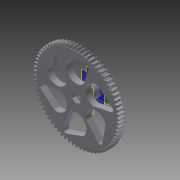
# Autodesk Inventor part: quarterinch-gear2
Saved by Autodesk Inventor 2014 (Build 180170000, 170)
## iProperties
Created: 2013-11-06
Part Number: quarterinch-gear2
Material: Generic
Document SubType Name: Modeling
Designer: stephen
Density: 1 g/cm^3
Appearance: Default
Author: stephen
Autodesk Inventor part; units mm, degrees
ref_plane "YZ Plane" through (0, 0, 0) normal (1, 0, 0) x (0, 1, 0)
ref_plane "XZ Plane" through (0, 0, 0) normal (0, 1, 0) x (-1, 0, 0)
ref_plane "XY Plane" through (0, 0, 0) normal (0, 0, 1) x (1, 0, 0)
ref_plane "Work Plane10" through (2.7665, 46.0619, 25.38) normal (0, 0, 1) x (1, 0, 0)
sketch "Sketch15" plane through (2.7665, 46.0619, 25.38) normal (0, 0, 1) x (1, 0, 0)
  line L0 (-0.1767, 42.3028) -> (0.1689, 42.3028)
  arc A0 (0.9579, 39.3583) -> (0.1689, 42.3028) centre (-2.8295, 39.9215) ccw
  line L1 (0.1689, 42.3028) -> (0.9579, 39.3583) construction
  arc A1 (-0.1767, 42.3028) -> (-0.9656, 39.3582) centre (2.8217, 39.9215) ccw
  line L2 (-3.968, 42.1167) -> (-3.6238, 42.1476)
  arc A2 (-2.5741, 39.2858) -> (-3.6238, 42.1476) centre (-6.3966, 39.5071) ccw
  line L3 (-3.6238, 42.1476) -> (-2.5741, 39.2858) construction
  arc A3 (-3.968, 42.1167) -> (-4.4898, 39.1132) centre (-0.7682, 40.0137) ccw
  line L4 (-7.7273, 41.5914) -> (-7.3873, 41.6531)
  arc A4 (-6.0852, 38.8969) -> (-7.3873, 41.6531) centre (-9.9122, 38.7747) ccw
  line L5 (-7.3873, 41.6531) -> (-6.0852, 38.8969) construction
  arc A5 (-7.7273, 41.5914) -> (-7.9778, 38.5532) centre (-4.3519, 39.7837) ccw
  line L6 (-11.4244, 40.7313) -> (-11.0913, 40.8233)
  arc A6 (-9.5474, 38.1948) -> (-11.0913, 40.8233) centre (-13.3481, 37.7301) ccw
  line L7 (-11.0913, 40.8233) -> (-9.5474, 38.1948) construction
  arc A7 (-11.4244, 40.7313) -> (-11.4015, 37.6829) centre (-7.9006, 39.2335) ccw
  line L8 (-15.0295, 39.5433) -> (-14.706, 39.6647)
  arc A8 (-12.9328, 37.1852) -> (-14.706, 39.6647) centre (-16.6764, 36.3817) ccw
  line L9 (-14.706, 39.6647) -> (-12.9328, 37.1852) construction
  arc A9 (-15.0295, 39.5433) -> (-14.7335, 36.5092) centre (-11.3856, 38.3673) ccw
  line L10 (-18.5137, 38.0368) -> (-18.2023, 38.1868)
  arc A10 (-16.2139, 35.8762) -> (-18.2023, 38.1868) centre (-19.8705, 34.7403) ccw
  line L11 (-18.2023, 38.1868) -> (-16.2139, 35.8762) construction
  arc A11 (-18.5137, 38.0368) -> (-17.9468, 35.0415) centre (-14.779, 37.1923) ccw
  line L12 (-21.8487, 36.2242) -> (-21.5521, 36.4014)
  arc A12 (-19.3646, 34.2784) -> (-21.5521, 36.4014) centre (-22.9046, 32.8193) ccw
  line L13 (-21.5521, 36.4014) -> (-19.3646, 34.2784) construction
  arc A13 (-21.8487, 36.2242) -> (-21.0157, 33.2917) centre (-18.0534, 35.7178) ccw
  line L14 (-25.0079, 34.1198) -> (-24.7283, 34.323)
  arc A14 (-22.3593, 32.4046) -> (-24.7283, 34.323) centre (-25.7543, 30.634) ccw
  line L15 (-24.7283, 34.323) -> (-22.3593, 32.4046) construction
  arc A15 (-25.0079, 34.1198) -> (-23.9153, 31.2738) centre (-21.1825, 33.9557) ccw
  line L16 (-27.9657, 31.7408) -> (-27.7055, 31.9681)
  arc A16 (-25.174, 30.2699) -> (-27.7055, 31.9681) centre (-28.3967, 28.2021) ccw
  line L17 (-27.7055, 31.9681) -> (-25.174, 30.2699) construction
  arc A17 (-27.9657, 31.7408) -> (-26.6224, 29.0042) centre (-24.1409, 31.9202) ccw
  line L18 (-30.6983, 29.1062) -> (-30.4595, 29.356)
  arc A18 (-27.7861, 27.8914) -> (-30.4595, 29.356) centre (-30.8104, 25.5431) ccw
  line L19 (-30.4595, 29.356) -> (-27.7861, 27.8914) construction
  arc A19 (-30.6983, 29.1062) -> (-29.1152, 26.501) centre (-26.9051, 29.6277) ccw
  line L20 (-33.1838, 26.2372) -> (-32.9683, 26.5074)
  arc A20 (-30.1744, 25.2884) -> (-32.9683, 26.5074) centre (-32.976, 22.6785) ccw
  line L21 (-32.9683, 26.5074) -> (-30.1744, 25.2884) construction
  arc A21 (-33.1838, 26.2372) -> (-31.3735, 23.7845) centre (-29.4526, 27.0967) ccw
  line L22 (-35.4021, 23.157) -> (-35.2117, 23.4454)
  arc A22 (-32.3197, 22.4818) -> (-35.2117, 23.4454) centre (-34.8761, 19.6312) ccw
  line L23 (-35.2117, 23.4454) -> (-32.3197, 22.4818) construction
  arc A23 (-35.4021, 23.157) -> (-33.3792, 20.8764) centre (-31.7629, 24.3475) ccw
  line L24 (-37.3354, 19.8904) -> (-37.1716, 20.1947)
  arc A24 (-34.2049, 19.4942) -> (-37.1716, 20.1947) centre (-36.4955, 16.4259) ccw
  line L25 (-37.1716, 20.1947) -> (-34.2049, 19.4942) construction
  arc A25 (-37.3354, 19.8904) -> (-35.1162, 17.8003) centre (-33.8176, 21.4023) ccw
  line L26 (-38.968, 16.4636) -> (-38.8322, 16.7814)
  arc A26 (-35.8146, 16.3496) -> (-38.8322, 16.7814) centre (-37.8209, 13.0884) ccw
  line L27 (-38.8322, 16.7814) -> (-35.8146, 16.3496) construction
  arc A27 (-38.968, 16.4636) -> (-36.5704, 14.5808) centre (-35.5999, 18.2847) ccw
  line L28 (-40.2869, 12.9043) -> (-40.1802, 13.2329)
  arc A28 (-37.136, 13.0734) -> (-40.1802, 13.2329) centre (-38.8419, 9.6454) ccw
  line L29 (-40.1802, 13.2329) -> (-37.136, 13.0734) construction
  arc A29 (-40.2869, 12.9043) -> (-37.7302, 11.244) centre (-37.0956, 15.02) ccw
  line L30 (-41.2815, 9.241) -> (-41.2046, 9.5779)
  arc A30 (-38.1584, 9.6919) -> (-41.2046, 9.5779) centre (-39.5502, 6.1248) ccw
  line L31 (-41.2046, 9.5779) -> (-38.1584, 9.6919) construction
  arc A31 (-41.2815, 9.241) -> (-38.5862, 7.8166) centre (-38.2927, 11.6343) ccw
  line L32 (-41.9437, 5.5034) -> (-41.8973, 5.8458)
  arc A32 (-38.8736, 6.2324) -> (-41.8973, 5.8458) centre (-39.94, 2.5549) ccw
  line L33 (-41.8973, 5.8458) -> (-38.8736, 6.2324) construction
  arc A33 (-41.9437, 5.5034) -> (-39.1316, 4.3263) centre (-39.1814, 8.1549) ccw
  line L34 (-42.2681, 1.7214) -> (-42.2526, 2.0666)
  arc A34 (-39.2757, 2.7227) -> (-42.2526, 2.0666) centre (-40.0082, -1.0355) ccw
  line L35 (-42.2526, 2.0666) -> (-39.2757, 2.7227) construction
  arc A35 (-42.2681, 1.7214) -> (-39.3618, 0.8012) centre (-39.7547, 4.6099) ccw
  line L36 (-42.2523, -2.0744) -> (-42.2678, -1.7292)
  arc A36 (-39.3617, -0.8089) -> (-42.2678, -1.7292) centre (-39.7543, -4.6177) ccw
  line L37 (-42.2678, -1.7292) -> (-39.3617, -0.8089) construction
  arc A37 (-42.2523, -2.0744) -> (-39.2752, -2.7304) centre (-40.0079, 1.0278) ccw
  line L38 (-41.8962, -5.8535) -> (-41.9426, -5.5111)
  arc A38 (-39.1307, -4.334) -> (-41.9426, -5.5111) centre (-39.1804, -8.1626) ccw
  line L39 (-41.9426, -5.5111) -> (-39.1307, -4.334) construction
  arc A39 (-41.8962, -5.8535) -> (-38.8723, -6.24) centre (-39.9389, -2.5626) ccw
  line L40 (-41.2029, -9.5855) -> (-41.2798, -9.2486)
  arc A40 (-38.5847, -7.8242) -> (-41.2798, -9.2486) centre (-38.2909, -11.6419) ccw
  line L41 (-41.2798, -9.2486) -> (-38.5847, -7.8242) construction
  arc A41 (-41.2029, -9.5855) -> (-38.1565, -9.6994) centre (-39.5484, -6.1324) ccw
  line L42 (-40.1777, -13.2403) -> (-40.2845, -12.9117)
  arc A42 (-37.728, -11.2514) -> (-40.2845, -12.9117) centre (-37.0932, -15.0274) ccw
  line L43 (-40.2845, -12.9117) -> (-37.728, -11.2514) construction
  arc A43 (-40.1777, -13.2403) -> (-37.1334, -13.0807) centre (-38.8395, -9.6528) ccw
  line L44 (-38.8292, -16.7885) -> (-38.965, -16.4708)
  arc A44 (-36.5676, -14.588) -> (-38.965, -16.4708) centre (-35.5968, -18.2919) ccw
  line L45 (-38.965, -16.4708) -> (-36.5676, -14.588) construction
  arc A45 (-38.8292, -16.7885) -> (-35.8114, -16.3566) centre (-37.8179, -13.0955) ccw
  line L46 (-37.1679, -20.2015) -> (-37.3317, -19.8972)
  arc A46 (-35.1127, -17.8072) -> (-37.3317, -19.8972) centre (-33.8139, -21.4091) ccw
  line L47 (-37.3317, -19.8972) -> (-35.1127, -17.8072) construction
  arc A47 (-37.1679, -20.2015) -> (-34.201, -19.5009) centre (-36.4918, -16.4328) ccw
  line L48 (-35.2074, -23.4519) -> (-35.3978, -23.1635)
  arc A48 (-33.3751, -20.883) -> (-35.3978, -23.1635) centre (-31.7586, -24.354) ccw
  line L49 (-35.3978, -23.1635) -> (-33.3751, -20.883) construction
  arc A49 (-35.2074, -23.4519) -> (-32.3153, -22.4882) centre (-34.8718, -19.6377) ccw
  line L50 (-32.9635, -26.5135) -> (-33.179, -26.2433)
  arc A50 (-31.3688, -23.7906) -> (-33.179, -26.2433) centre (-29.4477, -27.1028) ccw
  line L51 (-33.179, -26.2433) -> (-31.3688, -23.7906) construction
  arc A51 (-32.9635, -26.5135) -> (-30.1694, -25.2944) centre (-32.9711, -22.6845) ccw
  line L52 (-30.4541, -29.3616) -> (-30.693, -29.1118)
  arc A52 (-29.1099, -26.5067) -> (-30.693, -29.1118) centre (-26.8997, -29.6333) ccw
  line L53 (-30.693, -29.1118) -> (-29.1099, -26.5067) construction
  arc A53 (-30.4541, -29.3616) -> (-27.7806, -27.8969) centre (-30.805, -25.5487) ccw
  line L54 (-27.6996, -31.9733) -> (-27.9598, -31.7459)
  arc A54 (-26.6167, -29.0094) -> (-27.9598, -31.7459) centre (-24.1351, -31.9253) ccw
  line L55 (-27.9598, -31.7459) -> (-26.6167, -29.0094) construction
  arc A55 (-27.6996, -31.9733) -> (-25.1681, -30.2748) centre (-28.3908, -28.2072) ccw
  line L56 (-24.722, -34.3275) -> (-25.0016, -34.1244)
  arc A56 (-23.9092, -31.2786) -> (-25.0016, -34.1244) centre (-21.1762, -33.9603) ccw
  line L57 (-25.0016, -34.1244) -> (-23.9092, -31.2786) construction
  arc A57 (-24.722, -34.3275) -> (-22.3529, -32.409) centre (-25.748, -30.6386) ccw
  line L58 (-21.5454, -36.4054) -> (-21.8421, -36.2282)
  arc A58 (-21.0091, -33.2958) -> (-21.8421, -36.2282) centre (-18.0467, -35.7218) ccw
  line L59 (-21.8421, -36.2282) -> (-21.0091, -33.2958) construction
  arc A59 (-21.5454, -36.4054) -> (-19.3578, -34.2822) centre (-22.898, -32.8233) ccw
  line L60 (-18.1953, -38.1902) -> (-18.5067, -38.0402)
  arc A60 (-17.9399, -35.045) -> (-18.5067, -38.0402) centre (-14.772, -37.1956) ccw
  line L61 (-18.5067, -38.0402) -> (-17.9399, -35.045) construction
  arc A61 (-18.1953, -38.1902) -> (-16.2069, -35.8794) centre (-19.8635, -34.7437) ccw
  line L62 (-14.6987, -39.6674) -> (-15.0223, -39.546)
  arc A62 (-14.7263, -36.5121) -> (-15.0223, -39.546) centre (-11.3784, -38.3701) ccw
  line L63 (-15.0223, -39.546) -> (-14.7263, -36.5121) construction
  arc A63 (-14.6987, -39.6674) -> (-12.9254, -37.1878) centre (-16.6692, -36.3844) ccw
  line L64 (-11.0838, -40.8253) -> (-11.4169, -40.7334)
  arc A64 (-11.3941, -37.6852) -> (-11.4169, -40.7334) centre (-7.8931, -39.2355) ccw
  line L65 (-11.4169, -40.7334) -> (-11.3941, -37.6852) construction
  arc A65 (-11.0838, -40.8253) -> (-9.5399, -38.1967) centre (-13.3406, -37.7321) ccw
  line L66 (-7.3796, -41.6545) -> (-7.7196, -41.5928)
  arc A66 (-7.9702, -38.5548) -> (-7.7196, -41.5928) centre (-4.3443, -39.7851) ccw
  line L67 (-7.7196, -41.5928) -> (-7.9702, -38.5548) construction
  arc A67 (-7.3796, -41.6545) -> (-6.0776, -38.8981) centre (-9.9046, -38.7761) ccw
  line L68 (-3.616, -42.1483) -> (-3.9602, -42.1174)
  arc A68 (-4.4821, -39.114) -> (-3.9602, -42.1174) centre (-0.7605, -40.0144) ccw
  line L69 (-3.9602, -42.1174) -> (-4.4821, -39.114) construction
  arc A69 (-3.616, -42.1483) -> (-2.5663, -39.2863) centre (-6.3889, -39.5078) ccw
  line L70 (0.1767, -42.3028) -> (-0.1689, -42.3028)
  arc A70 (-0.9579, -39.3583) -> (-0.1689, -42.3028) centre (2.8295, -39.9215) ccw
  line L71 (-0.1689, -42.3028) -> (-0.9579, -39.3583) construction
  arc A71 (0.1767, -42.3028) -> (0.9656, -39.3582) centre (-2.8217, -39.9215) ccw
  line L72 (3.968, -42.1167) -> (3.6238, -42.1476)
  arc A72 (2.5741, -39.2858) -> (3.6238, -42.1476) centre (6.3966, -39.5071) ccw
  line L73 (3.6238, -42.1476) -> (2.5741, -39.2858) construction
  arc A73 (3.968, -42.1167) -> (4.4898, -39.1132) centre (0.7682, -40.0137) ccw
  line L74 (7.7273, -41.5914) -> (7.3873, -41.6531)
  arc A74 (6.0852, -38.8969) -> (7.3873, -41.6531) centre (9.9122, -38.7747) ccw
  line L75 (7.3873, -41.6531) -> (6.0852, -38.8969) construction
  arc A75 (7.7273, -41.5914) -> (7.9778, -38.5532) centre (4.3519, -39.7837) ccw
  line L76 (11.4244, -40.7313) -> (11.0913, -40.8233)
  arc A76 (9.5474, -38.1948) -> (11.0913, -40.8233) centre (13.3481, -37.7301) ccw
  line L77 (11.0913, -40.8233) -> (9.5474, -38.1948) construction
  arc A77 (11.4244, -40.7313) -> (11.4015, -37.6829) centre (7.9006, -39.2335) ccw
  line L78 (15.0295, -39.5433) -> (14.706, -39.6647)
  arc A78 (12.9328, -37.1852) -> (14.706, -39.6647) centre (16.6764, -36.3817) ccw
  line L79 (14.706, -39.6647) -> (12.9328, -37.1852) construction
  arc A79 (15.0295, -39.5433) -> (14.7335, -36.5092) centre (11.3856, -38.3673) ccw
  line L80 (18.5137, -38.0368) -> (18.2023, -38.1868)
  arc A80 (16.2139, -35.8762) -> (18.2023, -38.1868) centre (19.8705, -34.7403) ccw
  line L81 (18.2023, -38.1868) -> (16.2139, -35.8762) construction
  arc A81 (18.5137, -38.0368) -> (17.9468, -35.0415) centre (14.779, -37.1923) ccw
  line L82 (21.8487, -36.2242) -> (21.5521, -36.4014)
  arc A82 (19.3646, -34.2784) -> (21.5521, -36.4014) centre (22.9046, -32.8193) ccw
  line L83 (21.5521, -36.4014) -> (19.3646, -34.2784) construction
  arc A83 (21.8487, -36.2242) -> (21.0157, -33.2917) centre (18.0534, -35.7178) ccw
  line L84 (25.0079, -34.1198) -> (24.7283, -34.323)
  arc A84 (22.3593, -32.4046) -> (24.7283, -34.323) centre (25.7543, -30.634) ccw
  line L85 (24.7283, -34.323) -> (22.3593, -32.4046) construction
  arc A85 (25.0079, -34.1198) -> (23.9153, -31.2738) centre (21.1825, -33.9557) ccw
  line L86 (27.9657, -31.7408) -> (27.7055, -31.9681)
  arc A86 (25.174, -30.2699) -> (27.7055, -31.9681) centre (28.3967, -28.2021) ccw
  line L87 (27.7055, -31.9681) -> (25.174, -30.2699) construction
  arc A87 (27.9657, -31.7408) -> (26.6224, -29.0042) centre (24.1409, -31.9202) ccw
  line L88 (30.6983, -29.1062) -> (30.4595, -29.356)
  arc A88 (27.7861, -27.8914) -> (30.4595, -29.356) centre (30.8104, -25.5431) ccw
  line L89 (30.4595, -29.356) -> (27.7861, -27.8914) construction
  arc A89 (30.6983, -29.1062) -> (29.1152, -26.501) centre (26.9051, -29.6277) ccw
  line L90 (33.1838, -26.2372) -> (32.9683, -26.5074)
  arc A90 (30.1744, -25.2884) -> (32.9683, -26.5074) centre (32.976, -22.6785) ccw
  line L91 (32.9683, -26.5074) -> (30.1744, -25.2884) construction
  arc A91 (33.1838, -26.2372) -> (31.3735, -23.7845) centre (29.4526, -27.0967) ccw
  line L92 (35.4021, -23.157) -> (35.2117, -23.4454)
  arc A92 (32.3197, -22.4818) -> (35.2117, -23.4454) centre (34.8761, -19.6312) ccw
  line L93 (35.2117, -23.4454) -> (32.3197, -22.4818) construction
  arc A93 (35.4021, -23.157) -> (33.3792, -20.8764) centre (31.7629, -24.3475) ccw
  line L94 (37.3354, -19.8904) -> (37.1716, -20.1947)
  arc A94 (34.2049, -19.4942) -> (37.1716, -20.1947) centre (36.4955, -16.4259) ccw
  line L95 (37.1716, -20.1947) -> (34.2049, -19.4942) construction
  arc A95 (37.3354, -19.8904) -> (35.1162, -17.8003) centre (33.8176, -21.4023) ccw
  line L96 (38.968, -16.4636) -> (38.8322, -16.7814)
  arc A96 (35.8146, -16.3496) -> (38.8322, -16.7814) centre (37.8209, -13.0884) ccw
  line L97 (38.8322, -16.7814) -> (35.8146, -16.3496) construction
  arc A97 (38.968, -16.4636) -> (36.5704, -14.5808) centre (35.5999, -18.2847) ccw
  line L98 (40.2869, -12.9043) -> (40.1802, -13.2329)
  arc A98 (37.136, -13.0734) -> (40.1802, -13.2329) centre (38.8419, -9.6454) ccw
  line L99 (40.1802, -13.2329) -> (37.136, -13.0734) construction
  arc A99 (40.2869, -12.9043) -> (37.7302, -11.244) centre (37.0956, -15.02) ccw
  line L100 (41.2815, -9.241) -> (41.2046, -9.5779)
  arc A100 (38.1584, -9.6919) -> (41.2046, -9.5779) centre (39.5502, -6.1248) ccw
  line L101 (41.2046, -9.5779) -> (38.1584, -9.6919) construction
  arc A101 (41.2815, -9.241) -> (38.5862, -7.8166) centre (38.2927, -11.6343) ccw
  line L102 (41.9437, -5.5034) -> (41.8973, -5.8458)
  arc A102 (38.8736, -6.2324) -> (41.8973, -5.8458) centre (39.94, -2.5549) ccw
  line L103 (41.8973, -5.8458) -> (38.8736, -6.2324) construction
  arc A103 (41.9437, -5.5034) -> (39.1316, -4.3263) centre (39.1814, -8.1549) ccw
  line L104 (42.2681, -1.7214) -> (42.2526, -2.0666)
  arc A104 (39.2757, -2.7227) -> (42.2526, -2.0666) centre (40.0082, 1.0355) ccw
  line L105 (42.2526, -2.0666) -> (39.2757, -2.7227) construction
  arc A105 (42.2681, -1.7214) -> (39.3618, -0.8012) centre (39.7547, -4.6099) ccw
  line L106 (42.2523, 2.0744) -> (42.2678, 1.7292)
  arc A106 (39.3617, 0.8089) -> (42.2678, 1.7292) centre (39.7543, 4.6177) ccw
  line L107 (42.2678, 1.7292) -> (39.3617, 0.8089) construction
  arc A107 (42.2523, 2.0744) -> (39.2752, 2.7304) centre (40.0079, -1.0278) ccw
  line L108 (41.8962, 5.8535) -> (41.9426, 5.5111)
  arc A108 (39.1307, 4.334) -> (41.9426, 5.5111) centre (39.1804, 8.1626) ccw
  line L109 (41.9426, 5.5111) -> (39.1307, 4.334) construction
  arc A109 (41.8962, 5.8535) -> (38.8723, 6.24) centre (39.9389, 2.5626) ccw
  line L110 (41.2029, 9.5855) -> (41.2798, 9.2486)
  arc A110 (38.5847, 7.8242) -> (41.2798, 9.2486) centre (38.2909, 11.6419) ccw
  line L111 (41.2798, 9.2486) -> (38.5847, 7.8242) construction
  arc A111 (41.2029, 9.5855) -> (38.1565, 9.6994) centre (39.5484, 6.1324) ccw
  line L112 (40.1777, 13.2403) -> (40.2845, 12.9117)
  arc A112 (37.728, 11.2514) -> (40.2845, 12.9117) centre (37.0932, 15.0274) ccw
  line L113 (40.2845, 12.9117) -> (37.728, 11.2514) construction
  arc A113 (40.1777, 13.2403) -> (37.1334, 13.0807) centre (38.8395, 9.6528) ccw
  line L114 (38.8292, 16.7885) -> (38.965, 16.4708)
  arc A114 (36.5676, 14.588) -> (38.965, 16.4708) centre (35.5968, 18.2919) ccw
  line L115 (38.965, 16.4708) -> (36.5676, 14.588) construction
  arc A115 (38.8292, 16.7885) -> (35.8114, 16.3566) centre (37.8179, 13.0955) ccw
  line L116 (37.1679, 20.2015) -> (37.3317, 19.8972)
  arc A116 (35.1127, 17.8072) -> (37.3317, 19.8972) centre (33.8139, 21.4091) ccw
  line L117 (37.3317, 19.8972) -> (35.1127, 17.8072) construction
  arc A117 (37.1679, 20.2015) -> (34.201, 19.5009) centre (36.4918, 16.4328) ccw
  line L118 (35.2074, 23.4519) -> (35.3978, 23.1635)
  arc A118 (33.3751, 20.883) -> (35.3978, 23.1635) centre (31.7586, 24.354) ccw
  line L119 (35.3978, 23.1635) -> (33.3751, 20.883) construction
  arc A119 (35.2074, 23.4519) -> (32.3153, 22.4882) centre (34.8718, 19.6377) ccw
  line L120 (32.9635, 26.5135) -> (33.179, 26.2433)
  arc A120 (31.3688, 23.7906) -> (33.179, 26.2433) centre (29.4477, 27.1028) ccw
  line L121 (33.179, 26.2433) -> (31.3688, 23.7906) construction
  arc A121 (32.9635, 26.5135) -> (30.1694, 25.2944) centre (32.9711, 22.6845) ccw
  line L122 (30.4541, 29.3616) -> (30.693, 29.1118)
  arc A122 (29.1099, 26.5067) -> (30.693, 29.1118) centre (26.8997, 29.6333) ccw
  line L123 (30.693, 29.1118) -> (29.1099, 26.5067) construction
  arc A123 (30.4541, 29.3616) -> (27.7806, 27.8969) centre (30.805, 25.5487) ccw
  line L124 (27.6996, 31.9733) -> (27.9598, 31.7459)
  arc A124 (26.6167, 29.0094) -> (27.9598, 31.7459) centre (24.1351, 31.9253) ccw
  line L125 (27.9598, 31.7459) -> (26.6167, 29.0094) construction
  arc A125 (27.6996, 31.9733) -> (25.1681, 30.2748) centre (28.3908, 28.2072) ccw
  line L126 (24.722, 34.3275) -> (25.0016, 34.1244)
  arc A126 (23.9092, 31.2786) -> (25.0016, 34.1244) centre (21.1762, 33.9603) ccw
  line L127 (25.0016, 34.1244) -> (23.9092, 31.2786) construction
  arc A127 (24.722, 34.3275) -> (22.3529, 32.409) centre (25.748, 30.6386) ccw
  line L128 (21.5454, 36.4054) -> (21.8421, 36.2282)
  arc A128 (21.0091, 33.2958) -> (21.8421, 36.2282) centre (18.0467, 35.7218) ccw
  line L129 (21.8421, 36.2282) -> (21.0091, 33.2958) construction
  arc A129 (21.5454, 36.4054) -> (19.3578, 34.2822) centre (22.898, 32.8233) ccw
  line L130 (18.1953, 38.1902) -> (18.5067, 38.0402)
  arc A130 (17.9399, 35.045) -> (18.5067, 38.0402) centre (14.772, 37.1956) ccw
  line L131 (18.5067, 38.0402) -> (17.9399, 35.045) construction
  arc A131 (18.1953, 38.1902) -> (16.2069, 35.8794) centre (19.8635, 34.7437) ccw
  line L132 (14.6987, 39.6674) -> (15.0223, 39.546)
  arc A132 (14.7263, 36.5121) -> (15.0223, 39.546) centre (11.3784, 38.3701) ccw
  line L133 (15.0223, 39.546) -> (14.7263, 36.5121) construction
  arc A133 (14.6987, 39.6674) -> (12.9254, 37.1878) centre (16.6692, 36.3844) ccw
  line L134 (11.0838, 40.8253) -> (11.4169, 40.7334)
  arc A134 (11.3941, 37.6852) -> (11.4169, 40.7334) centre (7.8931, 39.2355) ccw
  line L135 (11.4169, 40.7334) -> (11.3941, 37.6852) construction
  arc A135 (11.0838, 40.8253) -> (9.5399, 38.1967) centre (13.3406, 37.7321) ccw
  line L136 (7.3796, 41.6545) -> (7.7196, 41.5928)
  arc A136 (7.9702, 38.5548) -> (7.7196, 41.5928) centre (4.3443, 39.7851) ccw
  line L137 (7.7196, 41.5928) -> (7.9702, 38.5548) construction
  arc A137 (7.3796, 41.6545) -> (6.0776, 38.8981) centre (9.9046, 38.7761) ccw
  line L138 (3.616, 42.1483) -> (3.9602, 42.1174)
  arc A138 (4.4821, 39.114) -> (3.9602, 42.1174) centre (0.7605, 40.0144) ccw
  line L139 (3.9602, 42.1174) -> (4.4821, 39.114) construction
  arc A139 (3.616, 42.1483) -> (2.5663, 39.2863) centre (6.3889, 39.5078) ccw
  line L140 (73.0043, -23.5061) -> (73.0043, 76.8994)
  line L141 (73.0043, -23.5061) -> (-27.4013, -23.5061) construction
  line L142 (12.7685, 31.9695) -> (7.0232, 15.0428)
  line L143 (-7.0232, 29.0892) -> (9.6761, 35.0189)
  arc A140 (-7.0232, 29.0892) -> (7.0232, 15.0428) centre (0, 22.066) ccw
  arc A141 (12.7685, 31.9695) -> (9.6761, 35.0189) centre (10.4835, 32.745) ccw
  line L144 (34.1169, 4.9001) -> (16.5854, 1.4124)
  arc A142 (21.7267, 20.6) -> (16.5854, 1.4124) centre (19.1561, 11.0062) ccw
  line L145 (21.7267, 20.6) -> (35.2117, 9.103)
  arc A143 (34.1169, 4.9001) -> (35.2117, 9.103) centre (33.6461, 7.2667) ccw
  line L146 (21.3176, -27.0693) -> (9.5313, -13.6305)
  arc A144 (28.719, -8.4891) -> (9.5313, -13.6305) centre (19.1252, -11.0598) ccw
  line L147 (28.719, -8.4891) -> (25.5047, -25.916)
  arc A145 (21.3176, -27.0693) -> (25.5047, -25.916) centre (23.1317, -25.4783) ccw
  line L148 (-12.7685, -31.9695) -> (-7.0232, -15.0428)
  arc A146 (7.0232, -29.0892) -> (-7.0232, -15.0428) centre (0, -22.066) ccw
  line L149 (7.0232, -29.0892) -> (-9.6761, -35.0189)
  arc A147 (-12.7685, -31.9695) -> (-9.6761, -35.0189) centre (-10.4835, -32.745) ccw
  line L150 (-34.0551, -4.9002) -> (-16.5236, -1.4124)
  arc A148 (-21.6649, -20.6001) -> (-16.5236, -1.4124) centre (-19.0942, -11.0062) ccw
  line L151 (-21.6649, -20.6001) -> (-35.1498, -9.103)
  arc A149 (-34.0551, -4.9002) -> (-35.1498, -9.103) centre (-33.5843, -7.2668) ccw
  line L152 (-21.2557, 27.0693) -> (-9.4695, 13.6304)
  arc A150 (-28.6572, 8.489) -> (-9.4695, 13.6304) centre (-19.0633, 11.0597) ccw
  line L153 (-28.6572, 8.489) -> (-25.4429, 25.9159)
  arc A151 (-21.2557, 27.0693) -> (-25.4429, 25.9159) centre (-23.0699, 25.4782) ccw
  line L154 (11.0838, 0) -> (38.8367, 0) construction
  line L155 (0, 0) -> (0, -16.4636)
  line L156 (0, 0) -> (9.5313, 0)
  line L157 (11.0838, 0) -> (9.4861, 0)
  line L158 (2.4848, 0) -> (0, 0)
  line L159 (0, 0) -> (0, -5.6488)
  line L160 (0, -11.1197) -> (0, -12.1337)
  arc A152 (-32.3153, -22.4882) -> (-31.3688, -23.7906) centre (0, 0) ccw
  arc A153 (-34.201, -19.5009) -> (-33.3751, -20.883) centre (0, 0) ccw
  arc A154 (-35.8114, -16.3566) -> (-35.1127, -17.8072) centre (0, 0) ccw
  arc A155 (-37.1334, -13.0807) -> (-36.5676, -14.588) centre (0, 0) ccw
  arc A156 (-38.8723, -6.24) -> (-38.5847, -7.8242) centre (0, 0) ccw
  arc A157 (-38.1565, -9.6994) -> (-37.728, -11.2514) centre (0, 0) ccw
  arc A158 (-39.2752, -2.7304) -> (-39.1307, -4.334) centre (0, 0) ccw
  arc A159 (-39.3618, 0.8012) -> (-39.3617, -0.8089) centre (0, 0) ccw
  arc A160 (-39.1316, 4.3263) -> (-39.2757, 2.7227) centre (0, 0) ccw
  arc A161 (-38.5862, 7.8166) -> (-38.8736, 6.2324) centre (0, 0) ccw
  arc A162 (-37.7302, 11.244) -> (-38.1584, 9.6919) centre (0, 0) ccw
  arc A163 (-36.5704, 14.5808) -> (-37.136, 13.0734) centre (0, 0) ccw
  arc A164 (-35.1162, 17.8003) -> (-35.8146, 16.3496) centre (0, 0) ccw
  arc A165 (-30.1694, -25.2944) -> (-29.1099, -26.5067) centre (0, 0) ccw
  arc A166 (-27.7806, -27.8969) -> (-26.6167, -29.0094) centre (0, 0) ccw
  arc A167 (-25.1681, -30.2748) -> (-23.9092, -31.2786) centre (0, 0) ccw
  arc A168 (-22.3529, -32.409) -> (-21.0091, -33.2958) centre (0, 0) ccw
  arc A169 (-19.3578, -34.2822) -> (-17.9399, -35.045) centre (0, 0) ccw
  arc A170 (-16.2069, -35.8794) -> (-14.7263, -36.5121) centre (0, 0) ccw
  arc A171 (-12.9254, -37.1878) -> (-11.3941, -37.6852) centre (0, 0) ccw
  arc A172 (-9.5399, -38.1967) -> (-7.9702, -38.5548) centre (0, 0) ccw
  arc A173 (-6.0776, -38.8981) -> (-4.4821, -39.114) centre (0, 0) ccw
  arc A174 (-2.5663, -39.2863) -> (-0.9579, -39.3583) centre (0, 0) ccw
  arc A175 (-33.3792, 20.8764) -> (-34.2049, 19.4942) centre (0, 0) ccw
  arc A176 (-31.3735, 23.7845) -> (-32.3197, 22.4818) centre (0, 0) ccw
  arc A177 (-29.1152, 26.501) -> (-30.1744, 25.2884) centre (0, 0) ccw
  arc A178 (-26.6224, 29.0042) -> (-27.7861, 27.8914) centre (0, 0) ccw
  arc A179 (-23.9153, 31.2738) -> (-25.174, 30.2699) centre (0, 0) ccw
  arc A180 (-21.0157, 33.2917) -> (-22.3593, 32.4046) centre (0, 0) ccw
  arc A181 (-17.9468, 35.0415) -> (-19.3646, 34.2784) centre (0, 0) ccw
  arc A182 (-14.7335, 36.5092) -> (-16.2139, 35.8762) centre (0, 0) ccw
  arc A183 (-11.4015, 37.6829) -> (-12.9328, 37.1852) centre (0, 0) ccw
  arc A184 (-7.9778, 38.5532) -> (-9.5474, 38.1948) centre (0, 0) ccw
  arc A185 (-4.4898, 39.1132) -> (-6.0852, 38.8969) centre (0, 0) ccw
  arc A186 (-0.9656, 39.3582) -> (-2.5741, 39.2858) centre (0, 0) ccw
  arc A187 (2.5663, 39.2863) -> (0.9579, 39.3583) centre (0, 0) ccw
  arc A188 (6.0776, 38.8981) -> (4.4821, 39.114) centre (0, 0) ccw
  arc A189 (9.5399, 38.1967) -> (7.9702, 38.5548) centre (0, 0) ccw
  arc A190 (12.9254, 37.1878) -> (11.3941, 37.6852) centre (0, 0) ccw
  arc A191 (16.2069, 35.8794) -> (14.7263, 36.5121) centre (0, 0) ccw
  arc A192 (19.3578, 34.2822) -> (17.9399, 35.045) centre (0, 0) ccw
  arc A193 (22.3529, 32.409) -> (21.0091, 33.2958) centre (0, 0) ccw
  arc A194 (25.1681, 30.2748) -> (23.9092, 31.2786) centre (0, 0) ccw
  arc A195 (27.7806, 27.8969) -> (26.6167, 29.0094) centre (0, 0) ccw
  arc A196 (30.1694, 25.2944) -> (29.1099, 26.5067) centre (0, 0) ccw
  arc A197 (32.3153, 22.4882) -> (31.3688, 23.7906) centre (0, 0) ccw
  arc A198 (34.201, 19.5009) -> (33.3751, 20.883) centre (0, 0) ccw
  arc A199 (35.8114, 16.3566) -> (35.1127, 17.8072) centre (0, 0) ccw
  arc A200 (37.1334, 13.0807) -> (36.5676, 14.588) centre (0, 0) ccw
  arc A201 (38.1565, 9.6994) -> (37.728, 11.2514) centre (0, 0) ccw
  arc A202 (38.8723, 6.24) -> (38.5847, 7.8242) centre (0, 0) ccw
  arc A203 (39.2752, 2.7304) -> (39.1307, 4.334) centre (0, 0) ccw
  arc A204 (39.3618, -0.8012) -> (39.3617, 0.8089) centre (0, 0) ccw
  arc A205 (39.1316, -4.3263) -> (39.2757, -2.7227) centre (0, 0) ccw
  arc A206 (38.5862, -7.8166) -> (38.8736, -6.2324) centre (0, 0) ccw
  arc A207 (37.7302, -11.244) -> (38.1584, -9.6919) centre (0, 0) ccw
  arc A208 (36.5704, -14.5808) -> (37.136, -13.0734) centre (0, 0) ccw
  arc A209 (35.1162, -17.8003) -> (35.8146, -16.3496) centre (0, 0) ccw
  arc A210 (33.3792, -20.8764) -> (34.2049, -19.4942) centre (0, 0) ccw
  arc A211 (31.3735, -23.7845) -> (32.3197, -22.4818) centre (0, 0) ccw
  arc A212 (29.1152, -26.501) -> (30.1744, -25.2884) centre (0, 0) ccw
  arc A213 (26.6224, -29.0042) -> (27.7861, -27.8914) centre (0, 0) ccw
  arc A214 (23.9153, -31.2738) -> (25.174, -30.2699) centre (0, 0) ccw
  arc A215 (21.0157, -33.2917) -> (22.3593, -32.4046) centre (0, 0) ccw
  arc A216 (17.9468, -35.0415) -> (19.3646, -34.2784) centre (0, 0) ccw
  arc A217 (14.7335, -36.5092) -> (16.2139, -35.8762) centre (0, 0) ccw
  arc A218 (11.4015, -37.6829) -> (12.9328, -37.1852) centre (0, 0) ccw
  arc A219 (7.9778, -38.5532) -> (9.5474, -38.1948) centre (0, 0) ccw
  arc A220 (0.9656, -39.3582) -> (2.5741, -39.2858) centre (0, 0) ccw
  arc A221 (4.4898, -39.1132) -> (6.0852, -38.8969) centre (0, 0) ccw
  dimension "d70" = 360
  dimension "d105" = 90
  constraints: 322 end point, 305 point on circle, 152 centre point, 4 perpendicular, 4 point on line, 3 horizontal, 2 collinear, 913 other
  measures "d105" angle of L141 L140
extrude "Extrusion18" add sketch "Sketch15" along normal blind 5.588
ref_plane "Work Plane8" through (2.7665, 46.0619, 14.665) normal (0, 0, -1) x (-1, 0, 0)
ref_plane "Work Plane11" through (2.7665, 46.0619, 14.665) normal (0, 0, -1) x (-1, 0, 0)
sketch "Sketch21" plane through (2.7665, 46.0619, 14.665) normal (0, 0, -1) x (-1, 0, 0)
  circle A0 centre (0, 0) radius 7.5 projected
  arc A1 (-26.2839, -1.3667) -> (-26.1961, -2.545) centre (0, 0) ccw projected
  circle A2 centre (0, 0) radius 7.5
  point P0 (2.7665, -46.0619)
  dimension "d114" = 15
  constraints: 1 centre point, 1 coincident, 1 concentric
  measures "d114" diameter of A0
extrude "Extrusion19" add sketch "Sketch21" against normal up to next
ref_plane "Work Plane12" through (2.7665, 46.0619, 14.665) normal (0, 0, -1) x (-1, 0, 0)
sketch "Sketch22" plane through (2.7665, 46.0619, 14.665) normal (0, 0, -1) x (-1, 0, 0)
  arc A0 (-26.2839, -1.3667) -> (-26.1961, -2.545) centre (0, 0) ccw projected
  circle A1 centre (0, 0) radius 7.5057
  point P0 (2.7665, -46.0619)
  dimension "d115" = 15.0114
  constraints: 1 centre point, 1 coincident
  measures "d115" diameter of A1
extrude "Extrusion20" add sketch "Sketch22" along normal blind 4.6
sketch "Sketch23" plane through (2.7665, 46.0619, 30.968) normal (0, 0, 1) x (1, 0, 0)
  arc A0 (2.5663, 39.2863) -> (0.9579, 39.3583) centre (0, 0) ccw projected
  line L0 (0, -4.792) -> (-4.15, -2.396)
  line L1 (-4.15, -2.396) -> (-4.15, 2.396)
  line L2 (-4.15, 2.396) -> (0, 4.792)
  line L3 (0, 4.792) -> (4.15, 2.396)
  line L4 (4.15, 2.396) -> (4.15, -2.396)
  line L5 (4.15, -2.396) -> (0, -4.792)
  point P0 (-2.7665, -46.0619)
  dimension "d118" = 8.3
  constraints: 12 end point, 1 coincident, 13 other
  measures "d118" distance between parallel lines of L4 L1
extrude "Extrusion21" cut sketch "Sketch23" against normal blind 4
ref_plane "Work Plane14" through (2.7665, 46.0619, 10.065) normal (0, 0, -1) x (-1, 0, 0)
sketch "Sketch24" plane through (2.7665, 46.0619, 10.065) normal (0, 0, -1) x (-1, 0, 0)
  circle A0 centre (0, 0) radius 7.5057 projected
  circle A1 centre (0, 0) radius 2.65
  point P0 (2.7665, -46.0619)
  dimension "d121" = 5.3
  constraints: 1 centre point, 1 coincident
  measures "d121" diameter of A1
extrude "Extrusion22" cut sketch "Sketch24" against normal through all contours A1
ref_plane "Work Plane13" through (2.7665, 46.0619, 10.065) normal (0, 0, -1) x (-1, 0, 0)
sketch "Sketch25" plane through (2.7665, 46.0619, 10.065) normal (0, 0, -1) x (-1, 0, 0)
  circle A0 centre (0, 0) radius 2.65 projected
  circle A1 centre (0, 0) radius 7.5057 projected
  circle A2 centre (0, 0) radius 4
  point P0 (2.7665, -46.0619)
  dimension "d124" = 8
  constraints: 1 centre point, 1 coincident
  measures "d124" diameter of A2
extrude "Extrusion23" add sketch "Sketch25" along normal blind 6 contours A2
body "Solid1"
